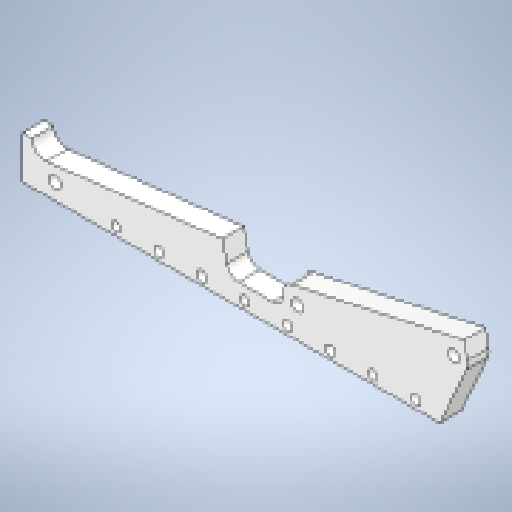
# Autodesk Inventor part: Uprights
Saved by Autodesk Inventor 2023.2 (Build 272271000, 271)
## iProperties
Created: 2024-01-11
Part Number: Uprights
Material: UHMW, White
Document SubType Name: Modeling
Designer: Nathan Cai
Mass: 10.4432 g
Surface Area: 60.6231 cm^2
Volume: 11.1098 cm^3
Density: 0.94 g/cm^3
Appearance: Smooth - White
Author: Nathan Cai
Autodesk Inventor part; units mm, degrees
ref_plane "YZ Plane" through (0, 0, 0) normal (1, 0, 0) x (0, 1, 0)
ref_plane "XZ Plane" through (0, 0, 0) normal (0, 1, 0) x (-1, 0, 0)
ref_plane "XY Plane" through (0, 0, 0) normal (0, 0, 1) x (1, 0, 0)
sketch "Sketch3" plane through (0, 0, 0) normal (0, 0, 1) x (1, 0, 0)
  line L0 (-48.8137, 10.438) -> (-52.9368, 29.0364) construction
  line L1 (-52.9368, 29.0364) -> (-59.1363, 27.662) construction
  line L2 (-59.1363, 27.662) -> (-55.0132, 9.0636) construction
  line L3 (-55.0132, 9.0636) -> (-48.8137, 10.438) construction
  line L4 (-48.8137, 10.438) -> (-59.1363, 27.662) construction
  line L5 (-52.9368, 29.0364) -> (-55.0132, 9.0636) construction
  circle A0 centre (-50.8753, 19.7372) radius 1.7526
  circle A1 centre (-59.1363, 27.662) radius 1.7526
  circle A2 centre (-55.0132, 9.0636) radius 1.7526
  line L6 (0, 0) -> (-127, 0)
  line L7 (0, 60.0769) -> (0, 0) construction
  line L8 (-44.6831, 6.4756) -> (-50.8679, 34.3732)
  line L9 (-50.8679, 34.3732) -> (-63.2669, 31.6244) construction
  line L10 (-63.2669, 31.6244) -> (-57.0821, 3.7268) construction
  line L11 (-57.0821, 3.7268) -> (-44.6831, 6.4756) construction
  line L12 (-44.6831, 6.4756) -> (-63.2669, 31.6244) construction
  line L13 (-50.8679, 34.3732) -> (-57.0821, 3.7268) construction
  line L14 (-45.2216, 8.9044) -> (-50.032, 30.6026)
  line L15 (-50.8679, 34.3732) -> (0, 45.6504) construction
  arc A3 (-128.0308, 9.4121) -> (-127, 0) centre (-127, 4.7625) ccw
  line L16 (-127, 0) -> (-127, 4.7625) construction
  line L17 (-128.0308, 9.4121) -> (-65.3965, 23.2978)
  line L18 (-9.6463, 43.5118) -> (0, 0)
  circle A4 centre (-127, 4.7625) radius 1.7526
  line L19 (-111.125, 0) -> (-12.7, 0) construction
  line L20 (-12.7, 0) -> (-12.7, 4.7625) construction
  line L21 (-12.7, 4.7625) -> (-111.125, 4.7625) construction
  line L22 (-111.125, 4.7625) -> (-111.125, 0) construction
  line L23 (-12.7, 2.3812) -> (-111.125, 2.3812) construction
  circle A5 centre (-108.7437, 2.3812) radius 1.4732
  circle A6 centre (-96.0437, 2.3812) radius 1.4732
  circle A7 centre (-83.3438, 2.3812) radius 1.4732
  circle A8 centre (-70.6437, 2.3812) radius 1.4732
  circle A9 centre (-57.9438, 2.3812) radius 1.4732
  circle A10 centre (-45.2438, 2.3812) radius 1.4732
  circle A11 centre (-32.5438, 2.3812) radius 1.4732
  circle A12 centre (-19.8438, 2.3812) radius 1.4732
  circle A13 centre (-8.5171, 19.3715) radius 1.7526
  line L24 (-55.0132, 9.0636) -> (-8.5171, 19.3715) construction
  line L25 (-53.9824, 4.414) -> (-8.0676, 14.593) construction
  line L26 (-5.5232, 24.9134) -> (-56.0439, 13.7132)
  arc A14 (-56.0439, 13.7132) -> (-53.9824, 4.414) centre (-55.0132, 9.0636) ccw construction
  line L27 (-5.5232, 24.9134) -> (-76.0422, 9.2797)
  line L28 (-76.0422, 9.2797) -> (-78.5057, 20.3916)
  line L29 (-78.5057, 20.3916) -> (-7.9866, 36.0253)
  line L30 (-7.9866, 36.0253) -> (-5.5232, 24.9134)
  line L31 (-50.5317, 18.1873) -> (-129.4495, 8.8468)
  line L32 (-59.1437, 13.026) -> (-76.0422, 13.026) construction
  line L33 (-76.0422, 13.026) -> (-76.0422, 6.35) construction
  line L34 (-76.0422, 6.35) -> (-59.1437, 6.35)
  line L35 (-59.1437, 6.35) -> (-59.1437, 13.026)
  arc A15 (-76.0422, 9.2797) -> (-72.3919, 6.35) centre (-72.3919, 10.0889) ccw
  line L36 (-127, 0) -> (-136.525, 0)
  line L37 (-136.525, 0) -> (-136.525, 12.7)
  line L38 (-136.525, 12.7) -> (-127, 12.7)
  line L39 (-127, 12.7) -> (-127, 0)
  arc A16 (-133.7857, 12.7) -> (-129.4495, 8.8468) centre (-129.9056, 12.7) ccw
  circle A17 centre (-8.5171, 19.3715) radius 4.1224
  line L40 (-12.7, 0) -> (-4.7567, 17.6823)
  point P0 (-53.975, 19.05)
  point P1 (-53.975, 19.05)
  point P2 (-53.975, 19.05)
  point P3 (-127, 0)
  point P4 (-46.7447, 15.7748)
  point P5 (-78.5057, 20.3916)
  point P6 (-77.3143, 15.0174)
  point P7 (-4.4924, 20.2638)
  dimension "d71" = 19.05
  dimension "d72" = 6.35
  dimension "d73" = 3.5052
  dimension "d74" = 3.5052
  dimension "d75" = 3.5052
  dimension "d76" = 127
  dimension "d77" = 19.05
  dimension "d78" = 12.5
  dimension "d91" = 12.7
  dimension "d92" = 28.575
  dimension "d93" = 53.975
  dimension "d98" = 9.525
  dimension "d107" = 3.5052
  dimension "d108" = 98.425
  dimension "d109" = 4.7625
  dimension "d110" = 15.875
  dimension "d111" = 2.9464
  dimension "d112" = 2.3813
  dimension "d115" = 12.7
  dimension "d120" = 3.5052
  dimension "d127" = 3.175
  dimension "d129" = 6.75
  dimension "d135" = 47.625
  dimension "d136" = 72.2313
  dimension "d137" = 4.7625
  dimension "d138" = 6.35
  dimension "d139" = 9.525
  dimension "d140" = 12.7
  constraints: 84 end point, 17 centre point, 17 parallel, 15 point on line, 9 midpoint, 9 point on circle, 7 tangent, 6 perpendicular, 5 horizontal, 4 coincident, 2 vertical, 1 collinear, 1 line through centre, 19 other
  measures "d71" distance between parallel lines of L3 L1
  measures "d72" distance between parallel lines of L2 L0
  measures "d73" diameter of A0
  measures "d74" diameter of A1
  measures "d75" diameter of A2
  measures "d76" distance of L6.end L6.start
  measures "d77" distance from line of L6 point (-53.975, 19.05)
  measures "d78" angle of L6 L3
  measures "d91" distance between parallel lines of L10 L8
  measures "d92" distance between parallel lines of L11 L9
  measures "d93" distance from line of L7 point (-53.975, 19.05)
  measures "d98" diameter of A3
  measures "d107" diameter of A4
  measures "d108" distance of L21.end L20.end
  measures "d109" distance of L20.end L19.end
  measures "d110" distance between parallel lines of L16 L22
  measures "d111" diameter of A5
  measures "d112" distance from line of A5.centre L22
  measures "d115" distance of A5.centre A6.centre
  measures "d120" diameter of A13
  measures "d127" distance from line of L31.start L27
  measures "d129" angle of L6 L31
  measures "d135" distance from line of L2 L24.end
  measures "d136" distance between parallel lines of L30 L28
  measures "d137" radius of A14
  measures "d138" distance between parallel lines of L6 L34
  measures "d139" distance of L37.end L38.end
  measures "d140" distance of L36.end L37.end
extrude "Extrusion3" add sketch "Sketch3" along normal blind 6.35 contours L28 A15 L34 L35 L27 L26 L18 A17 L40 L6 L39 A4 L31 | L39 A4 A3 L31 | A3 L36 L37 L38 A16 | A17
extrude "Extrusion4" cut sketch "Sketch3" along normal through all contours A13
fillet "Fillet7" radius 3.175 2 edges at (-59.1437, 13.026, 3.175) (-59.1437, 6.35, 3.175)
equation "\"Angle_Mount\" = 105deg"
equation "\"Rail_Offset\" = 36.5125"
body "Solid3"
